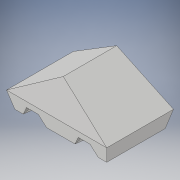
# Autodesk Inventor part: tesla v1
Saved by Autodesk Inventor 2018 (Build 220112000, 112)
## iProperties
Created: 2020-01-07
Part Number: tesla v1
Material: Generic
Document SubType Name: Modeling
Designer: AOFUser
Density: 1 g/cm^3
Appearance: Default
Author: AOFUser
Autodesk Inventor part; units mm, degrees
ref_plane "YZ Plane" through (0, 0, 0) normal (1, 0, 0) x (0, 1, 0)
ref_plane "XZ Plane" through (0, 0, 0) normal (0, 1, 0) x (-1, 0, 0)
ref_plane "XY Plane" through (0, 0, 0) normal (0, 0, 1) x (1, 0, 0)
sketch "Sketch1" plane through (0, 0, 0) normal (0, 1, 0) x (-1, 0, 0)
  line L0 (0, 0) -> (-76.2, 0)
  line L1 (-76.2, 0) -> (-76.2, -50.8)
  line L2 (-76.2, -50.8) -> (0, -50.8)
  line L3 (0, -50.8) -> (0, 0)
  dimension "d0" = 76.2
  dimension "d1" = 50.8
  constraints: 8 end point, 2 parallel, 1 horizontal, 1 perpendicular
  measures "d0" distance of L2.end L1.end
  measures "d1" distance of L1.end L0.end
extrude "Extrusion1" add sketch "Sketch1" along normal blind 12.7
chamfer "Chamfer1" distance 12.7 distance2 3.175 1 edges at (38.1, 0, -50.8) measured on face at (50.8, 4.2333, -50.8)
chamfer "Chamfer2" distance 12.7 distance2 3.175 1 edges at (38.1, 0, 0) measured on face at (25.4, 4.2333, 0)
chamfer "Chamfer3" distance 12.7 distance2 3.175 1 edges at (76.2, 0, -25.4) measured on face at (76.2, 8.4663, -32.8085)
chamfer "Chamfer4" distance 12.7 distance2 3.175 1 edges at (0, 0, -25.4) measured on face at (0, 8.4663, -17.9915)
sketch "Sketch2" plane through (0, 12.7, 0) normal (0, 1, 0) x (1, 0, 0)
  line L0 (0, 50.8) -> (3.175, 47.625) projected
  line L1 (0, 0) -> (76.2, 0) projected
  line L2 (0, 50.8) -> (76.2, 50.8)
  line L3 (76.2, 50.8) -> (76.2, 0)
  line L4 (76.2, 0) -> (0, 0)
  line L5 (0, 0) -> (0, 50.8)
  constraints: 8 end point, 2 parallel, 1 horizontal, 1 perpendicular
extrude "Extrusion2" add sketch "Sketch2" along normal blind 25.4
chamfer "Chamfer5" distance 5.08 distance2 25.4 1 edges at (38.1, 38.1, 0) measured on face at (25.4, 38.1, -33.8667)
chamfer "Chamfer6" distance 5.08 distance2 25.4 1 edges at (38.1, 38.1, -50.8) measured on face at (50.8, 38.1, -20.32)
chamfer "Chamfer7" distance 38.1 distance2 25.4 1 edges at (0, 38.1, -25.4) measured on face at (50.8, 38.1, -18.6267)
chamfer "Chamfer8" distance 38.1 distance2 25.4 1 edges at (76.2, 38.1, -25.4) measured on face at (50.8, 38.1, -32.1733)
sketch "Sketch6" plane through (3.175, 0, -3.175) normal (0, -0.2425, 0.9701) x (1, 0, 0)
  line L0 (0, 0) -> (69.85, 0) projected
  line L1 (0, 0) -> (15.24, 0)
  line L2 (15.24, 0) -> (24.13, 0)
  line L3 (69.85, 0) -> (69.85, -10.7807) projected
  line L4 (69.85, 0) -> (54.61, 0)
  line L5 (54.61, 0) -> (45.72, 0)
  line L6 (24.13, 0) -> (19.685, -7.699)
  line L7 (19.685, -7.699) -> (10.795, -7.699)
  line L8 (10.795, -7.699) -> (6.35, 0)
  line L9 (6.35, 0) -> (10.795, 7.699)
  line L10 (10.795, 7.699) -> (19.685, 7.699)
  line L11 (19.685, 7.699) -> (24.13, 0)
  line L12 (45.72, 0) -> (50.165, 7.699)
  line L13 (50.165, 7.699) -> (59.055, 7.699)
  line L14 (59.055, 7.699) -> (63.5, 0)
  line L15 (63.5, 0) -> (59.055, -7.699)
  line L16 (59.055, -7.699) -> (50.165, -7.699)
  line L17 (50.165, -7.699) -> (45.72, 0)
  point P0 (-3.175, 0.7701)
  dimension "d34" = 15.24
  dimension "d35" = 8.89
  dimension "d36" = 15.24
  dimension "d37" = 8.89
  constraints: 32 end point, 4 point on line, 2 coincident, 26 other
  measures "d34" distance of L0.start L1.end
  measures "d35" distance of L1.end L2.end
  measures "d36" distance of L0.end L4.end
  measures "d37" distance of L4.end L5.end
extrude "Extrusion3" cut sketch "Sketch6" against normal blind 7.62 contours L9 L10 L11 L0 | L0 L6 L7 L8
sketch "Sketch7" plane through (0, 12.7, 0) normal (0, -0.2425, 0.9701) x (1, 0, 0)
  line L0 (27.305, -13.0909) -> (73.025, -13.0909) projected
  line L1 (73.025, -13.0909) -> (57.785, -13.0909)
  line L2 (57.785, -13.0909) -> (48.895, -13.0909)
  line L3 (48.895, -13.0909) -> (53.34, -5.3919)
  line L4 (53.34, -5.3919) -> (62.23, -5.3919)
  line L5 (62.23, -5.3919) -> (66.675, -13.0909)
  line L6 (66.675, -13.0909) -> (62.23, -20.7898)
  line L7 (62.23, -20.7898) -> (53.34, -20.7898)
  line L8 (53.34, -20.7898) -> (48.895, -13.0909)
  point P0 (0, -12.3208)
  dimension "d40" = 15.24
  dimension "d41" = 8.89
  constraints: 16 end point, 2 point on line, 1 coincident, 13 other
  measures "d40" distance of L0.end L1.end
  measures "d41" distance of L1.end L2.end
extrude "Extrusion4" cut sketch "Sketch7" against normal blind 7.62
sketch "Sketch8" plane through (73.025, 0, -47.625) normal (0, -0.2425, -0.9701) x (-1, 0, 0)
  line L0 (69.85, 0) -> (69.85, -10.7807) projected
  line L1 (69.85, 0) -> (54.61, 0)
  line L2 (0, 0) -> (69.85, 0) projected
  line L3 (54.61, 0) -> (45.72, 0)
  line L4 (45.72, 0) -> (50.165, 7.699)
  line L5 (50.165, 7.699) -> (59.055, 7.699)
  line L6 (59.055, 7.699) -> (63.5, 0)
  line L7 (63.5, 0) -> (59.055, -7.699)
  line L8 (59.055, -7.699) -> (50.165, -7.699)
  line L9 (50.165, -7.699) -> (45.72, 0)
  point P0 (73.025, -11.5508)
  dimension "d44" = 15.24
  dimension "d45" = 8.89
  constraints: 16 end point, 2 point on line, 1 coincident, 13 other
  measures "d44" distance of L0.start L1.end
  measures "d45" distance of L1.end L3.end
extrude "Extrusion5" cut sketch "Sketch8" against normal blind 7.62
body "Solid1"
